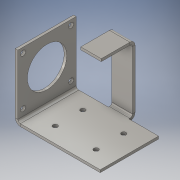
# Autodesk Inventor part: MotorClamptwo
Saved by Autodesk Inventor 2016 (Build 200138000, 138)
## iProperties
Created: 2017-02-14
Part Number: MotorClamptwo
Material: Steel, Mild
Document SubType Name: Sheet Metal
Designer: Evan Phil George
Density: 7.85 g/cm^3
Sheet Metal Rule: 2.5mmSS
Appearance: Semi-Polished
Flat Pattern Width: 15.431 cm
Flat Pattern Length: 14.2155 cm
Flat Pattern Area: 219.359 cm^2
Sheet Metal Width: 154.310 mm
Sheet Metal Length: 142.155 mm
Sheet Metal Area: 21935.880 mm^2
Author: Evan Phil George
Autodesk Inventor part; units mm, degrees
ref_plane "YZ Plane" through (0, 0, 0) normal (1, 0, 0) x (0, 1, 0)
ref_plane "XZ Plane" through (0, 0, 0) normal (0, 1, 0) x (-1, 0, 0)
ref_plane "XY Plane" through (0, 0, 0) normal (0, 0, 1) x (1, 0, 0)
sketch "Sketch1" plane through (0, 0, 0) normal (0, 1, 0) x (-1, 0, 0)
  line L0 (39, -28.5) -> (-39, -28.5)
  line L1 (-39, -28.5) -> (-39, 28.5)
  line L2 (-39, 28.5) -> (39, 28.5)
  line L3 (39, 28.5) -> (39, -28.5)
  line L4 (39, -28.5) -> (-39, 28.5) construction
  line L5 (-39, -28.5) -> (39, 28.5) construction
  point P0 (0, 0)
  dimension "d0" = 78
  dimension "d1" = 57
  measures "d0" distance of L1.end L2.end
  measures "d1" distance of L0.end L1.end
extrude "Plate1" add sketch "Sketch1" along normal blind 2.5
sketch "Sketch2" plane through (-41.5, 5, 28.5) normal (-1, 0, 0) x (0, -1, 0)
  line L0 (0, -57) -> (0, 0)
  line L1 (0, 0) -> (-58.5, 0)
  line L2 (-58.5, 0) -> (-58.5, -57)
  line L3 (-58.5, -57) -> (0, -57)
  constraints: 6 end point, 1 horizontal, 1 perpendicular, 1 vertical
edge flange "Flange1" height 63.5 angle 90 thickness 2.5 bend radius 2.5 thickness toward (-1, 0, 0) relief tear relief width 2.5 relief depth 1.25 edges at (-39, 2.5, 0) wall of the first edge with corners at (-41.5, 5, -28.5) (-41.5, 5, 28.5) (-41.5, 63.5, 28.5) (-41.5, 63.5, -28.5)
bend "Bend1"
corner "Corner1"
sketch "Sketch3" plane through (-41.5, 63.5, 28.5) normal (1, 0, 0) x (0, 0, -1)
  line L0 (57, 0) -> (57, -58.5) projected
  line L1 (0, 0) -> (57, 0)
  line L2 (57, 0) -> (57, -57)
  line L3 (57, -57) -> (0, -57)
  line L4 (0, -57) -> (0, 0)
  line L5 (0, 0) -> (57, -57)
  circle A0 centre (28.5, -28.5) radius 19.25
  line L6 (0, 0) -> (5, 0)
  line L7 (57, 0) -> (0, 0) projected
  line L8 (5, 0) -> (5, -5)
  line L9 (57, 0) -> (52, 0)
  line L10 (52, 0) -> (52, -5)
  line L11 (57, -57) -> (52, -57)
  line L12 (52, -57) -> (52, -52)
  line L13 (0, -57) -> (5, -57)
  line L14 (5, -57) -> (5, -52)
  circle A1 centre (5, -52) radius 2.5
  circle A2 centre (52, -52) radius 2.5
  circle A3 centre (52, -5) radius 2.5
  circle A4 centre (5, -5) radius 2.5
  point P0 (28.5, -63.5)
  dimension "d13" = 57
  dimension "d14" = 38.5
  dimension "d15" = 5
  dimension "d16" = 5
  dimension "d17" = 5
  dimension "d18" = 5
  dimension "d19" = 5
  dimension "d20" = 5
  dimension "d21" = 5
  dimension "d22" = 5
  dimension "d23" = 5
  dimension "d24" = 5
  dimension "d25" = 5
  dimension "d26" = 5
  constraints: 26 end point, 7 point on line, 5 centre point, 4 coincident, 3 perpendicular, 2 parallel, 1 horizontal, 1 midpoint
  measures "d13" distance of L1.end L2.end
  measures "d14" diameter of A0
  measures "d15" distance of L1.start L6.end
  measures "d16" distance of L6.end L8.end
  measures "d17" distance of L1.end L9.end
  measures "d18" distance of L9.end L10.end
  measures "d19" distance of L2.end L11.end
  measures "d20" distance of L11.end L12.end
  measures "d21" distance of L3.end L13.end
  measures "d22" distance of L13.end L14.end
  measures "d23" diameter of A1
  measures "d24" diameter of A2
  measures "d25" diameter of A3
  measures "d26" diameter of A4
extrude "Cut1" cut sketch "Sketch3" against normal blind 2.5 contours A2 L12 L5 | L5 A2 | A2 L5 L12 | A4 L5 L8 | L8 L5 A4 | L5 A4 | A0 L5 | L5 A0 | A1 | A3
sketch "Sketch4" plane through (39, 0, -28.5) normal (0, 0, -1) x (-1, 0, 0)
  line L0 (39, 0) -> (29, 0)
  line L1 (78, 0) -> (0, 0) projected
  line L2 (29, 0) -> (29, 2.5)
  line L3 (78, 2.5) -> (0, 2.5) projected
  line L4 (29, 2.5) -> (49, 2.5)
  line L5 (49, 2.5) -> (49, 0)
  line L6 (49, 0) -> (29, 0)
  line L7 (29, 0) -> (29, 2.5)
  dimension "d29" = 10
  dimension "d30" = 20
  constraints: 12 end point, 3 point on line, 2 parallel, 2 perpendicular, 1 horizontal
  measures "d29" distance of L0.start L0.end
  measures "d30" distance of L5.end L6.end
extrude "Extrusion1" add sketch "Sketch4" along normal blind 1
sketch "Sketch5" plane through (-10, 5, -32) normal (0, 0, -1) x (-1, 0, 0)
  line L0 (-20, 0) -> (0, 0)
  line L1 (0, 0) -> (0, 57)
  line L2 (0, 57) -> (-20, 57)
  line L3 (-20, 57) -> (-20, 0)
  constraints: 6 end point, 1 horizontal, 1 perpendicular, 1 vertical
edge flange "Flange2" height 62 angle 90 thickness 2.5 bend radius 2.5 thickness toward (0, 0, -1) relief tear relief width 2.5 relief depth 1.25 edges at (0, 2.5, -29.5) wall of the first edge with corners at (10, 5, -32) (-10, 5, -32) (-10, 62, -32) (10, 62, -32)
bend "Bend2"
corner "Corner2"
sketch "Sketch6" plane through (-10, 64.5, -29.5) normal (0, 1, 0) x (-1, 0, 0)
  line L0 (-20, 0) -> (0, 0)
  line L1 (0, 0) -> (0, 28)
  line L2 (0, 28) -> (-20, 28)
  line L3 (-20, 28) -> (-20, 0)
  constraints: 6 end point, 1 horizontal, 1 perpendicular, 1 vertical
edge flange "Flange3" height 33 angle 90 thickness 2.5 bend radius 2.5 thickness toward (0, 1, 0) relief tear relief width 2.5 relief depth 1.25 edges at (0, 62, -32) wall of the first edge with corners at (10, 64.5, -29.5) (-10, 64.5, -29.5) (-10, 64.5, -1.5) (10, 64.5, -1.5)
bend "Bend3"
corner "Corner3"
sketch "Sketch7" plane through (0, 2.5, 0) normal (0, 1, 0) x (1, 0, 0)
  line L0 (39, -28.5) -> (-39, -28.5) projected
  line L1 (0, -28.5) -> (0, -13.5)
  line L2 (0, -13.5) -> (20, -13.5)
  line L3 (0, -13.5) -> (-20, -13.5)
  circle A0 centre (-20, -13.5) radius 2.25
  circle A1 centre (20, -13.5) radius 2.25
  line L4 (0, -13.5) -> (0, 13.5)
  line L5 (0, 13.5) -> (20, 13.5)
  line L6 (0, 13.5) -> (-20, 13.5)
  circle A2 centre (-20, 13.5) radius 2.25
  circle A3 centre (20, 13.5) radius 2.25
  point P0 (0, 0)
  dimension "d53" = 15
  dimension "d54" = 20
  dimension "d55" = 20
  dimension "d56" = 4.5
  dimension "d57" = 4.5
  dimension "d58" = 27
  dimension "d59" = 20
  dimension "d60" = 20
  dimension "d61" = 4.5
  dimension "d62" = 4.5
  constraints: 12 end point, 4 centre point, 4 coincident, 3 perpendicular, 2 horizontal, 1 midpoint, 1 vertical
  measures "d53" distance of L1.start L1.end
  measures "d54" distance of L1.end L2.end
  measures "d55" distance of L1.end L3.end
  measures "d56" diameter of A0
  measures "d57" diameter of A1
  measures "d58" distance of L1.end L4.end
  measures "d59" distance of L4.end L5.end
  measures "d60" distance of L4.end L6.end
  measures "d61" diameter of A2
  measures "d62" diameter of A3
extrude "Cut2" cut sketch "Sketch7" against normal blind 2.5
equation "\"d27\" = Thickness"
equation "\"d63\" = Thickness"
equation "\"d3\" = BendReliefWidth"
equation "\"d4\" = BendReliefDepth"
equation "\"d5\" = MinimumRemnant"
equation "\"d6\" = BendRadius"
equation "\"d9\" = BendRadius"
equation "\"d10\" = CornerReliefSize"
equation "\"d11\" = GapSize"
equation "\"d12\" = JacobiRadiusSize"
equation "\"d33\" = BendReliefWidth"
equation "\"d34\" = BendReliefDepth"
equation "\"d35\" = MinimumRemnant"
equation "\"d36\" = BendRadius"
equation "\"d39\" = BendRadius"
equation "\"d40\" = CornerReliefSize"
equation "\"d41\" = GapSize"
equation "\"d42\" = JacobiRadiusSize"
equation "\"d43\" = BendReliefWidth"
equation "\"d44\" = BendReliefDepth"
equation "\"d45\" = MinimumRemnant"
equation "\"d46\" = BendRadius"
equation "\"d49\" = BendRadius"
equation "\"d50\" = CornerReliefSize"
equation "\"d51\" = GapSize"
equation "\"d52\" = JacobiRadiusSize"
equation "\"BendRadius\" = Thickness"
equation "\"BendReliefWidth\" = Thickness"
equation "\"BendReliefDepth\" = 0.5 * Thickness"
equation "\"MinimumRemnant\" = 2 * Thickness"
equation "\"TransitionRadius\" = BendRadius"
equation "\"JacobiRadiusSize\" = BendRadius"
equation "\"GapSize\" = Thickness"
equation "\"d2\" = BendRadius"
equation "\"Thickness\" = 2.5"
equation "\"CornerReliefSize\" = 10"
body "Solid1"
